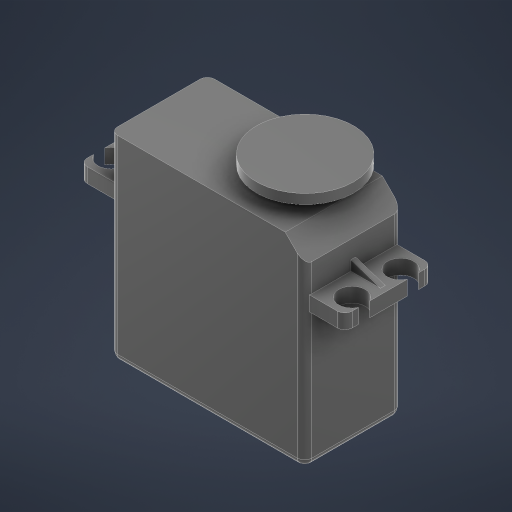
# Autodesk Inventor part: LDX-335MG_Servo_15kg_cm
Saved by Autodesk Inventor 2023 (Build 270158000, 158)
## iProperties
Created: 2023-02-24
Part Number: LDX-335MG_Servo_15kg_cm
Material: Steel
Document SubType Name: Modeling
Designer: roota
Density: 7.85 g/cm^3
Appearance: Smooth - Black
Author: roota
Autodesk Inventor part; units mm, degrees
ref_plane "YZ Plane" through (0, 0, 0) normal (1, 0, 0) x (0, 1, 0)
ref_plane "XY Plane" through (0, 0, 0) normal (0, 0, 1) x (1, 0, 0)
sketch "Sketch1" plane through (0, 0, 0) normal (0, 1, 0) x (-1, 0, 0)
  line L0 (30.1, 10) -> (-9.9, 10)
  line L1 (-9.9, 10) -> (-9.9, -10)
  line L2 (-9.9, -10) -> (30.1, -10)
  line L3 (30.1, -10) -> (30.1, 10)
  line L4 (30.1, 10) -> (-9.9, -10) construction
  line L5 (-9.9, 10) -> (30.1, -10) construction
  point P0 (0, 0)
  point P1 (10.1, 0)
  dimension "d0" = 40
  dimension "d1" = 20
  dimension "d2" = 9.9
  constraints: 12 end point, 2 midpoint, 2 parallel, 1 horizontal, 1 horizontal alignment, 1 perpendicular
  measures "d0" distance of L2.end L1.end
  measures "d1" distance of L1.end L0.end
  measures "d2" distance from line of point (0, 0) L1
extrude "Extrusion1" add sketch "Sketch1" along normal blind 40.5
ref_plane "Work Plane1" through (0, 27.8, 0) normal (0, 1, 0) x (-1, 0, 0)
sketch "Sketch2" plane through (0, 27.8, 0) normal (0, 1, 0) x (-1, 0, 0)
  line L0 (37.35, -9) -> (-17.15, -9)
  line L1 (-17.15, -9) -> (-17.15, 9)
  line L2 (-17.15, 9) -> (37.35, 9)
  line L3 (37.35, 9) -> (37.35, -9)
  circle A0 centre (-14.65, 5) radius 2.75
  circle A1 centre (-14.65, -5) radius 2.75
  circle A2 centre (34.85, -5) radius 2.75
  circle A3 centre (34.85, 5) radius 2.75
  line L4 (30.1, -10) -> (30.1, 10) projected
  line L5 (-9.9, 10) -> (-9.9, -10) projected
  point P0 (0, 0)
  point P1 (-9.9, -9)
  point P2 (-9.9, 9)
  point P3 (-17.15, 6.1456)
  point P4 (-17.15, 3.8544)
  point P5 (-17.15, -3.8544)
  point P6 (-17.15, -6.1456)
  point P7 (30.1, 9)
  point P8 (30.1, -9)
  point P9 (37.35, -6.1456)
  point P10 (37.35, -3.8544)
  point P11 (37.35, 3.8544)
  point P12 (37.35, 6.1456)
  dimension "d6" = 18
  dimension "d7" = 9
  dimension "d8" = 54.5
  dimension "d9" = 5.5
  dimension "d10" = 49.5
  dimension "d11" = 10
  dimension "d12" = 2.5
  dimension "d13" = 5
  dimension "d14" = 7.25
  dimension "d15" = 7.25
  constraints: 8 end point, 4 centre point, 3 equal radius, 2 horizontal alignment, 2 parallel, 2 vertical alignment, 1 horizontal, 1 perpendicular
  measures "d6" distance of L0.end L1.end
  measures "d7" distance from line of point (0, 0) L2
  measures "d8" distance of L1.end L2.end
  measures "d9" diameter of A0
  measures "d10" distance of A0.centre A3.centre
  measures "d11" distance of A1.centre A0.centre
  measures "d12" distance from line of L1 A0.centre
  measures "d13" vertical distance of point (0, 0) A1.centre
  measures "d14" distance between parallel lines of L4 L3
  measures "d15" distance between parallel lines of L1 L5
extrude "Extrusion2" add sketch "Sketch2" along normal blind 3 contours L0 L4 L2 L3 A3 A2 | L0 L1 A1 A0 L2 L5
chamfer "Chamfer1" distance 4 angle 45 1 edges at (9.9, 40.5, 0)
fillet "Fillet1" radius 1.5 12 edges at (-30.1, 20.25, 10) (-30.1, 20.25, -10) (9.9, 18.25, -10) (9.9, 18.25, 10) (17.15, 29.3, -9) (17.15, 29.3, 9) (-37.35, 29.3, 9) (-37.35, 29.3, -9) (-10.1, 0, 10) (-30.1, 0, 0) (-10.1, 0, -10) (9.9, 0, 0)
sketch "Sketch3" plane through (0, 40.5, 0) normal (0, 1, 0) x (1, 0, 0)
  circle A0 centre (0, 0) radius 2
  dimension "d19" = 4
  constraints: 1 centre point, 1 coincident
  measures "d19" diameter of A0
extrude "Extrusion3" add sketch "Sketch3" along normal blind 1
sketch "Sketch4" plane through (0, 41.5, 0) normal (0, 1, 0) x (1, 0, 0)
  circle A0 centre (0, 0) radius 4
  dimension "d22" = 8
  constraints: 1 centre point, 1 coincident
  measures "d22" diameter of A0
extrude "Extrusion4" add sketch "Sketch4" along normal blind 3
sketch "Sketch5" plane through (0, 44.5, 0) normal (0, 1, 0) x (1, 0, 0)
  circle A0 centre (0, 0) radius 10
  dimension "d25" = 20
  constraints: 1 centre point, 1 coincident
  measures "d25" diameter of A0
extrude "Extrusion5" add sketch "Sketch5" along normal blind 2
sketch "Sketch6" plane through (0, 0, 0) normal (0, 0, 1) x (1, 0, 0)
  line L0 (10.0603, 32.7866) -> (15.6122, 30.9286)
  line L1 (-30.2038, 33.1105) -> (-35.8273, 30.9286)
  point P0 (0, 0)
  constraints: 4 end point
extrude "Rib1" add sketch "Sketch6" along normal mid plane 1 rib yes fills toward (-32.9974, 31.9729) open curves L1
extrude "Rib2" add sketch "Sketch6" along normal mid plane 1 rib yes fills toward (12.8203, 31.8102) open curves L0
equation "\"d7\" = 0.5 * d6"
equation "\"d12\" = -0.5 * d10 + 0.5 * d8"
equation "\"d13\" = 0.5 * d11"
equation "\"d14\" = d15"
body "Solid1"
